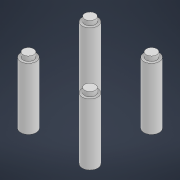
# Autodesk Inventor part: 110033226_ipt_26_騎樓梁架
Saved by Autodesk Inventor 2022 (Build 260153000, 153)
## iProperties
Created: 2022-06-24
Part Number: 110033226_ipt_26_騎樓梁架
Material: 一般
Document SubType Name: Modeling
Designer: User
Density: 1 g/cm^3
Appearance: 預設
Author: User
Autodesk Inventor part; units mm, degrees
ref_plane "YZ Plane" through (0, 0, 0) normal (1, 0, 0) x (0, 1, 0)
ref_plane "XZ Plane" through (0, 0, 0) normal (0, 1, 0) x (-1, 0, 0)
ref_plane "XY Plane" through (0, 0, 0) normal (0, 0, 1) x (1, 0, 0)
sketch "草圖1" plane through (0, 0, 0) normal (0, 1, 0) x (-1, 0, 0)
  circle A0 centre (10, 10) radius 1.7
  circle A1 centre (10, 10) radius 2.5
  line L0 (12.5, 12.5) -> (-12.5, 12.5)
  line L1 (-12.5, 12.5) -> (-12.5, -12.5)
  line L2 (-12.5, -12.5) -> (12.5, -12.5)
  line L3 (12.5, -12.5) -> (12.5, 12.5)
  point P0 (0, 0)
  point P1 (12.5, 0)
  point P2 (0, -12.5)
  dimension "d0" = 3.4
  dimension "d1" = 5
  dimension "d11" = 25
  dimension "d12" = 25
  dimension "d13" = 2.5
  dimension "d14" = 2.5
  constraints: 8 end point, 2 centre point, 2 midpoint, 2 parallel, 1 coincident, 1 horizontal, 1 horizontal alignment, 1 perpendicular, 1 vertical alignment
  measures "d0" diameter of A0
  measures "d1" diameter of A1
  measures "d11" distance of L2.end L1.end
  measures "d12" distance of L1.end L0.end
  measures "d13" distance from line of L3 A0.centre
  measures "d14" distance from line of L0 A0.centre
extrude "擠出1" add sketch "草圖1" along normal blind 20 contours A0 | A1
extrude "擠出2" cut sketch "草圖1" along normal blind 1.5 contours A0
sketch "草圖2" plane through (-10, 20, 10) normal (0, 1, 0) x (1, 0, 0)
  circle A0 centre (0, 0) radius 1.7 projected
  point P0 (10, 10)
extrude "擠出3" add sketch "草圖2" along normal blind 1.5
pattern_circular "環形陣列1" count 4 over 360 about axis through (0, -10, 0) along (0, 1, 0) of "擠出1", "擠出3", "擠出2"
